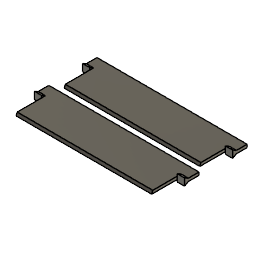
card-shuffler (Autodesk Fusion 360 archive; units mm, degrees)
design "card-shuffler-gates"
part number: 2026-07-29-22-33-21-616
part number: 2026-07-29-22-39-06-031
Autodesk Fusion 360 part; units mm, degrees
note: some values were not read from the file. Set by a fixed rule: which face or edge a step refers to.
(part 1 of 12)
sketch "Sketch1" plane through (0, 0, 0) normal (0, 0, 1) x (1, 0, 0)
  line L0 (0, 0) -> (93, 0)
  line L1 (93, 0) -> (93, -17.5)
  line L2 (93, -17.5) -> (0, -17.5)
  line L3 (0, -17.5) -> (0, 0)
  line L4 (93, 0) -> (98, 0)
  line L5 (93, -5) -> (93, 0)
  line L6 (0, 0) -> (-5, 0)
  line L7 (0, -15.5) -> (0, 0)
  line L8 (-5, 0) -> (98, 0)
  line L9 (98, 0) -> (98, 10)
  line L10 (98, 10) -> (-5, 10)
  line L11 (-5, 10) -> (-5, 0)
  line L12 (0, -15.5) -> (93, -15.5)
  line L13 (93, -15.5) -> (93, 10)
  line L14 (93, 10) -> (0, 10)
  line L15 (0, 10) -> (0, -15.5)
  dimension "d1" = 93
  dimension "d17" = 10
  dimension "d22" = 15.5
  dimension "d23" = 2
  constraint horizontal L0
  constraint vertical L1
  constraint horizontal L2
  constraint vertical L3
  constraint coincident L0.start L3.end
  constraint horizontal L4
  constraint vertical L5
  constraint horizontal L6
  constraint vertical L7
  constraint horizontal L8
  constraint vertical L9
  constraint horizontal L10
  constraint vertical L11
  constraint horizontal L12
  constraint vertical L13
  constraint horizontal L14
  constraint vertical L15
  constraint coincident L10 L13.end
  measures "d1" distance of L0.start L0.end
  measures "d17" distance of L6.end L10.end
  measures "d22" distance of L8 L12
  measures "d23" distance of L2 L12
extrude "Extrude1" add sketch "Sketch1" along normal blind 2 contours L6 L8 L10 L11 L15 | L4 L8 L9 L10 L13 makes body 1 at (-1.6667, 3.3333, 0) makes body 2 at (96.3333, 3.3333, 0)
extrude "Extrude3" add sketch "Sketch1" along normal blind 2 contours L0 L8 L10 L13 L14 L15 | L0 L1 L3 L5 L7 L8 L12 L13 L15 | L1 L2 L3 L12 bodies 1 2
sketch "Sketch3" plane through (0, 0, 0) normal (1, 0, 0) x (0, -1, 0)
  line L0 (-9, -5) -> (5, -5)
  line L1 (5, -5) -> (5, -2)
  line L2 (-9, -2) -> (16.216, -2) construction
  line L3 (5, -5) -> (10.1764, -5) construction
  line L4 (-9, -2) -> (-9, -5)
  line L5 (5, -2) -> (-9, -2)
  line L6 (0, 0) -> (17.5, 0)
  line L7 (17.5, 0) -> (17.5, -2)
  line L8 (17.5, -2) -> (0, -2)
  line L9 (17.5, 0) -> (16.7721, -2)
  line L10 (17.5, 0) -> (9.1284, 0) construction
  line L11 (0, -2) -> (0, 0)
  dimension "d16" = 110
  constraint horizontal L2
  constraint coincident L2.start L4.start
  constraint horizontal L3
  constraint coincident L0.end L1.start
  constraint horizontal L10
  constraint coincident L6.end L7.start
  constraint coincident L2 L9.end
  measures "d16" angle of L9 L10
extrude "Extrude2" cut sketch "Sketch3" along normal blind 95 contours L7 L8 L9 bodies 1
sketch "Sketch4" plane through (-5, 0, 0) normal (-1, 0, 0) x (0, -1, 0)
  line L0 (-10, 0) -> (0, 0)
  line L1 (0, 0) -> (0, 2)
  line L2 (0, 2) -> (-10, 2)
  line L3 (-10, 2) -> (-10, 0)
  line L4 (0, -1.5) -> (0, 3.5)
  line L5 (0, 3.5) -> (-4.3301, 1)
  line L6 (-4.3301, 1) -> (0, -1.5)
  point P0 (-1.4434, 1)
sketch "Sketch5" plane through (98, 0, 0) normal (1, 0, 0) x (0, 1, 0)
  line L0 (0, 0) -> (10, 0)
  line L1 (10, 0) -> (10, 2)
  line L2 (10, 2) -> (0, 2)
  line L3 (0, 2) -> (0, 0)
  line L4 (0, -1.5) -> (4.3301, 1)
  line L5 (4.3301, 1) -> (0, 3.5)
  line L6 (0, 3.5) -> (0, -1.5)
  point P0 (1.4434, 1)
extrude "Extrude4" add sketch "Sketch5" against normal blind 5 contours L0 L4 L6 | L2 L5 L6 bodies 1
extrude "Extrude5" add sketch "Sketch4" against normal blind 5 contours L0 L4 L6 | L2 L4 L5 bodies 1
copy_body "Body->Comp1" bodies 1 removing the originals makes body 3 in component "Component"
component "Component" placed x (1, 0, 0) y (0, 1, 0) z (0, 0, 1) at (0, 0, 0)
component "Component" placed x (1, 0, 0) y (0, 1, 0) z (0, 0, 1) at (0, 33, 0)
equation "d16 = 90 deg + 20 deg"

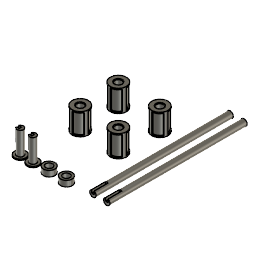
design "card-shuffler-wheels-and-shaft"
part number: 2026-07-30-19-48-15-416
part number: 2026-07-31-16-18-04-707
part number: 2026-07-31-16-25-10-615
part number: 2026-07-31-16-25-10-619
part number: 2026-08-15-23-04-46-105
part number: 2026-08-15-23-04-46-110
part number: 2026-08-17-15-33-29-178
Autodesk Fusion 360 part; units mm, degrees
sketch "Sketch4" plane through (0, 0, 0) normal (0, 0, 1) x (1, 0, 0)
  circle A0 centre (0, 0) radius 6
  circle A1 centre (0, 0) radius 7
  circle A2 centre (35, 0) radius 2.8
  circle A3 centre (0, 0) radius 7.5
  circle A4 centre (35, 0) radius 2.9
  line L0 (0, 0) -> (7, 0)
  line L1 (0, 0) -> (2.8348, 6.4003)
  line L2 (0, 0) -> (-7, 0) construction
  line L3 (0, 0) -> (-6.4003, 2.8348)
  line L4 (0, 0) -> (0, 7)
  line L5 (0, 0) -> (-2.8348, -6.4003)
  line L6 (0, 0) -> (-7, 0)
  line L7 (0, 0) -> (6.4003, -2.8348)
  line L8 (0, 0) -> (0, -7)
  circle A5 centre (0, -45) radius 5
  circle A6 centre (0, -45) radius 2.925
  circle A7 centre (-40, -45) radius 5
  line L9 (38, 1) -> (32, 1)
  line L10 (32, 1) -> (32, -1)
  line L11 (32, -1) -> (38, -1)
  line L12 (38, -1) -> (38, 1)
  line L13 (38, 1) -> (32, -1) construction
  line L14 (32, 1) -> (38, -1) construction
  line L15 (31.9, -1.1) -> (38.1, -1.1)
  line L16 (38.1, -1.1) -> (38.1, 1.1)
  line L17 (38.1, 1.1) -> (31.9, 1.1)
  line L18 (31.9, 1.1) -> (31.9, -1.1)
  line L19 (35, 1.1) -> (35, -1.1)
  line L20 (35.1, 1.1) -> (35.1, -1.1)
  point P0 (35, 0)
  dimension "d20" = 12
  dimension "d33" = 5.6
  dimension "d36" = 1
  dimension "d37" = 15
  dimension "d42" = 5.8
  dimension "d44" = 113.889
  dimension "d46" = 360
  dimension "d49" = 5.85
  dimension "d52" = 10
  dimension "d58" = 6
  dimension "d59" = 2
  dimension "d62" = 0.1
  constraint coincident A0.centre A1.centre
  constraint concentric A2 A4
  constraint coincident A1 L0.end
  constraint horizontal L0
  constraint horizontal L2
  constraint coincident A1 L1.end
  constraint concentric A5 A6
  constraint horizontal L9
  constraint perpendicular L9 L10
  constraint parallel L9 L11
  constraint parallel L10 L12
  constraint coincident L13 P0
  constraint coincident L14 P0
  constraint coincident P0 A2.centre
  constraint midpoint L17 L19.start
  constraint midpoint L15 L19.end
  constraint coincident L17 L20.start
  constraint coincident L15 L20.end
  constraint perpendicular L15 L20
  measures "d20" diameter of A0
  measures "d33" diameter of A2
  measures "d36" distance of A0 A1
  measures "d37" diameter of A3
  measures "d42" diameter of A4
  measures "d44" angle of L1 L2
  measures "d49" diameter of A6
  measures "d52" diameter of A7
  measures "d58" distance of L10.end L11.end
  measures "d59" distance of L9.end L10.end
extrude "Extrude3" add sketch "Sketch4" along normal blind 19 contours A0 L0 L1 | A0 L0 L7 | A0 L1 L4 | A0 L7 L8 | A0 L3 L6 | A0 L3 L4 | A0 L5 L8 | A0 L5 L6 makes body 1
sketch "Sketch5" plane through (0, 0, 19) normal (0, 0, 1) x (-1, 0, 0)
  circle A0 centre (0, 0) radius 6
  circle A1 centre (0, 0) radius 7
  circle A2 centre (0, 0) radius 2.925
  dimension "d24" = 14
  dimension "d29" = 5.85
  constraint coincident A0.centre A1.centre
  measures "d24" diameter of A1
  measures "d29" diameter of A2
extrude "Extrude5" add sketch "Sketch5" against normal blind 1 contours A1 bodies 1
extrude "Extrude4" add sketch "Sketch4" along normal blind 1 contours A0 A1 L0 L7 | A0 A1 L0 L1 | A0 A1 L1 L4 | A0 A1 L7 L8 | A0 A1 L3 L4 | A0 A1 L5 L8 | A0 A1 L3 L6 | A0 A1 L5 L6 bodies 1
extrude "Extrude6" cut sketch "Sketch5" against normal blind 19 contours A2 bodies 1
chamfer "Chamfer1" distance 0.5 angle 45 2 edges at (2.7271, 1.0577, 0) (2.7271, -1.0577, 19) on bodies 1
extrude "Extrude9" add sketch "Sketch4" along normal blind 19 contours A0 A1 L0 L7 | A0 A1 L1 L4 | A0 A1 L5 L8 | A0 A1 L3 L6 bodies 1
copy_body "Body->Comp2" bodies 1 removing the originals makes body 2 in component "Component"
extrude "Extrude7" add sketch "Sketch4" along normal blind 119 separate body contours A2 L9 L11 L20 | A2 L9 L17 L20 | A2 L11 L15 L20 | A2 L17 | L9 L11 L19 L20 | L9 L17 L19 L20 | A2 L15 | L11 L15 L19 L20 | A2 L9 L17 L19 | A2 L9 L11 L19 | A2 L11 L15 L19 makes body 3
extrude "Extrude13" cut sketch "Sketch4" along normal blind 12 contours L9 L11 L19 L20 | L9 L17 L19 L20 | L11 L15 L19 L20 | A2 L9 L17 L19 | A2 L9 L11 L19 | A2 L11 L15 L19 bodies 3
copy_body "CopyPasteBodies1" bodies 3 makes body 4
move_body "Move1" bodies 4 to x (1, 0, 0) y (0, 1, 0) z (0, 0, 1) at (-12, 0, 0)
copy_body "Body->Comp3" bodies 3 removing the originals makes body 5 in component "Component'"
copy_body "Body->Comp4" bodies 4 removing the originals makes body 6 in component "Component''"
move_body "Move1'" bodies 6 to x (1, 0, 0) y (0, 0, -1) z (0, 1, 0) at (0, -45, 3) in component "Component''"
move_body "Move1''" bodies 5 to x (1, 0, 0) y (0, 0, -1) z (0, 1, 0) at (0, -45, 3) in component "Component'"
extrude "Extrude10" add sketch "Sketch4" along normal blind 5 separate body contours A5 makes body 7
copy_body "CopyPasteBodies3" bodies 7 makes body 8
move_body "Move4" bodies 8 to x (1, 0, 0) y (0, 1, 0) z (0, 0, 1) at (-15, 0, 0)
copy_body "Body->Comp7" bodies 8 removing the originals makes body 9 in component "Component'''"
copy_body "Body->Comp8" bodies 7 removing the originals makes body 10 in component "Component''''"
extrude "Extrude11" add sketch "Sketch4" along normal blind 1 separate body contours A7 makes body 11
sketch "Sketch6" plane through (0, 0, 1) normal (0, 0, 1) x (-1, 0, 0)
  circle A0 centre (40, 45) radius 5
  circle A1 centre (40, 45) radius 2.8
  line L0 (37, 44) -> (43, 44)
  line L1 (43, 44) -> (43, 46)
  line L2 (43, 46) -> (37, 46)
  line L3 (37, 46) -> (37, 44)
  line L4 (37, 44) -> (43, 46) construction
  line L5 (43, 44) -> (37, 46) construction
  line L6 (40, 44) -> (40, 46)
  line L7 (39.9, 44) -> (39.9, 46)
  point P0 (40, 45)
  dimension "d55" = 5.6
  constraint concentric A0 A1
  constraint horizontal L0
  constraint perpendicular L0 L1
  constraint parallel L0 L2
  constraint parallel L1 L3
  constraint coincident L4 P0
  constraint coincident L5 P0
  constraint coincident P0 A0.centre
  constraint midpoint L0 L6.start
  constraint midpoint L2 L6.end
  constraint coincident L0 L7.start
  constraint coincident L2 L7.end
  constraint perpendicular L2 L7
  measures "d55" diameter of A1
extrude "Extrude12" add sketch "Sketch6" along normal blind 20 contours A1 L2 | A1 L0 | A1 L0 L2 L7 bodies 11
extrude "Extrude14" add sketch "Sketch6" along normal blind 8 contours A1 L0 L2 L6 bodies 11
copy_body "Body->Comp9" bodies 11 removing the originals makes body 12 in component "Component'''''"
component "Component" placed x (1, 0, 0) y (0, 1, 0) z (0, 0, 1) at (0, 0, 0)
component "Component" placed x (1, 0, 0) y (0, 1, 0) z (0, 0, 1) at (-33, 0, 0)
component "Component" placed x (1, 0, 0) y (0, 1, 0) z (0, 0, 1) at (-34, 34, 0)
component "Component" placed x (1, 0, 0) y (0, 1, 0) z (0, 0, 1) at (2, 34, 0)
component "Component'" placed x (0, 0, -1) y (0, 1, 0) z (1, 0, 0) at (31.9518, 0, 37.9518)
component "Component''" placed x (0, 0, -1) y (0, 1, 0) z (1, 0, 0) at (19.9518, 0, 25.9518)
component "Component'''" placed x (1, 0, 0) y (0, 1, 0) z (0, 0, 1) at (0, 0, 0)
component "Component''''" placed x (1, 0, 0) y (0, 1, 0) z (0, 0, 1) at (0, 0, 0)
component "Component'''''" placed x (1, 0, 0) y (0, 1, 0) z (0, 0, 1) at (0, 0, 0)
component "Component'''''" placed x (1, 0, 0) y (0, 1, 0) z (0, 0, 1) at (11, 0, 0)
equation "d34 = 93 mm + 20 mm + 6 mm"
equation "d44 = 180 deg - 66.11051484 deg"

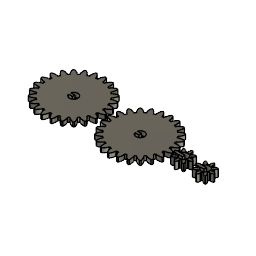
design "card-shuffler-middle-gears"
part number: 2026-08-17-02-18-25-515
part number: 2026-08-18-19-56-53-081
part number: 2026-08-18-20-31-36-499
Autodesk Fusion 360 part; units mm, degrees
sketch "Sketch1" plane through (0, 0, 0) normal (0, 0, 1) x (1, 0, 0) in component "Component"
  spline S0 degree 5 poles (4.4841, -1.024) (4.4842, -1.0241) (4.4844, -1.0241) (4.4848, -1.0242) (4.4853, -1.0243) (4.486, -1.0244) (4.4869, -1.0246) (4.4879, -1.0248) (4.489, -1.025) (4.4903, -1.0252) (4.4916, -1.0254) (4.4931, -1.0257) (4.4947, -1.0259) (4.4963, -1.0262) (4.4981, -1.0264) (4.5, -1.0267) (4.502, -1.027) (4.5042, -1.0272) (4.5064, -1.0275) (4.5087, -1.0278) (4.5111, -1.0281) (4.5136, -1.0284) (4.5162, -1.0287) (4.5189, -1.0289) (4.5218, -1.0292) (4.5247, -1.0295) (4.5277, -1.0297) (4.5308, -1.03) (4.534, -1.0302) (4.5372, -1.0305) (4.5406, -1.0307) (4.5441, -1.0309) (4.5476, -1.0311) (4.5513, -1.0313) (4.555, -1.0315) (4.5588, -1.0317) (4.5627, -1.0319) (4.5667, -1.032) (4.5708, -1.0321) (4.575, -1.0322) (4.5792, -1.0323) (4.5835, -1.0324) (4.5879, -1.0325) (4.5924, -1.0325) (4.597, -1.0325) (4.6016, -1.0325) (4.6064, -1.0325) (4.6111, -1.0324) (4.616, -1.0324) (4.621, -1.0323) (4.626, -1.0322) (4.6311, -1.032) (4.6363, -1.0319) (4.6415, -1.0317) (4.6468, -1.0315) (4.6522, -1.0312) (4.6577, -1.031) (4.6632, -1.0307) (4.6688, -1.0303) (4.6745, -1.03) (4.6802, -1.0296) (4.686, -1.0292) (4.6919, -1.0288) (4.6978, -1.0283) (4.7038, -1.0278) (4.7099, -1.0272) (4.716, -1.0267) (4.7222, -1.0261) (4.7285, -1.0255) (4.7348, -1.0248) (4.7412, -1.0241) (4.7476, -1.0234) (4.7541, -1.0226) (4.7607, -1.0218) (4.7673, -1.021) (4.774, -1.0201) (4.7807, -1.0192) (4.7875, -1.0182) (4.7944, -1.0173) (4.8013, -1.0162) (4.8083, -1.0152) (4.8153, -1.0141) (4.8224, -1.013) (4.8295, -1.0118) (4.8367, -1.0106) (4.8439, -1.0093) (4.8512, -1.0081) (4.8585, -1.0067) (4.8659, -1.0054) (4.8734, -1.004) (4.8809, -1.0025) (4.8884, -1.001) (4.896, -0.9995) (4.9037, -0.9979) (4.9114, -0.9963) (4.9191, -0.9947) (4.9269, -0.993) (4.9347, -0.9912) (4.9426, -0.9894) (4.9505, -0.9876) (4.9585, -0.9858) (4.9665, -0.9838) (4.9746, -0.9819) (4.9827, -0.9799) (4.9908, -0.9778) (4.999, -0.9757) (5.0073, -0.9736) (5.0155, -0.9714) (5.0239, -0.9692) (5.0322, -0.9669) (5.0406, -0.9646) (5.0491, -0.9623) (5.0576, -0.9599) (5.0661, -0.9574) (5.0746, -0.9549) (5.0832, -0.9524) (5.0919, -0.9498) (5.1005, -0.9471) (5.1092, -0.9444) (5.118, -0.9417) (5.1268, -0.9389) (5.1356, -0.9361) (5.1444, -0.9332) (5.1533, -0.9303) (5.1623, -0.9273) (5.1712, -0.9243) (5.1802, -0.9212) (5.1892, -0.9181) (5.1983, -0.9149) (5.2074, -0.9117) (5.2165, -0.9084) (5.2256, -0.9051) (5.2348, -0.9017) (5.244, -0.8983) (5.2533, -0.8948) (5.2626, -0.8913) (5.2719, -0.8877) (5.2812, -0.8841) (5.2905, -0.8804) (5.2999, -0.8767) (5.3094, -0.8729) (5.3188, -0.8691) (5.3283, -0.8652) (5.3378, -0.8613) (5.3473, -0.8573) (5.3568, -0.8533) (5.3664, -0.8492) (5.376, -0.8451) (5.3856, -0.8409) (5.3953, -0.8367) (5.4049, -0.8324) (5.4146, -0.8281) (5.4244, -0.8237) (5.4341, -0.8192) (5.4439, -0.8147) (5.4537, -0.8102) (5.4635, -0.8056) (5.4733, -0.8009) (5.4831, -0.7962) (5.493, -0.7915) (5.5029, -0.7867) (5.5128, -0.7818) (5.5227, -0.7769) (5.5327, -0.7719) (5.5426, -0.7669) (5.5526, -0.7618) (5.5626, -0.7567) (5.5726, -0.7515) (5.5827, -0.7463) (5.5927, -0.741) (5.6028, -0.7356) (5.6129, -0.7302) (5.623, -0.7248) (5.6331, -0.7193) (5.6432, -0.7137) (5.6534, -0.7081) (5.6636, -0.7024) (5.6737, -0.6967) (5.6839, -0.6909) (5.6941, -0.6851) (5.7043, -0.6792) (5.7146, -0.6733) (5.7248, -0.6673) (5.7351, -0.6613) (5.7453, -0.6552) (5.7556, -0.649) (5.7659, -0.6428) (5.7762, -0.6365) (5.7865, -0.6302) (5.7968, -0.6239) (5.8071, -0.6174) (5.8175, -0.611) (5.8278, -0.6044) (5.8382, -0.5978) (5.8485, -0.5912) (5.8589, -0.5845) (5.8693, -0.5777) (5.8797, -0.5709) (5.8901, -0.5641) (5.9005, -0.5572) (5.9109, -0.5502) (5.9213, -0.5432) (5.9317, -0.5361) (5.9421, -0.529) (5.9525, -0.5218) (5.963, -0.5145) (5.9734, -0.5072) (5.9839, -0.4999) (5.9943, -0.4925) (6.0048, -0.485) (6.0152, -0.4775) (6.0257, -0.4699) (6.0361, -0.4623) (6.0466, -0.4546) (6.057, -0.4469) (6.0675, -0.4391) (6.078, -0.4313) (6.0884, -0.4234) (6.0989, -0.4154) (6.1094, -0.4074) (6.1199, -0.3993) (6.1303, -0.3912) (6.1408, -0.383) (6.1513, -0.3748) (6.1617, -0.3665) (6.1722, -0.3582) (6.1827, -0.3498) (6.1931, -0.3414) (6.2036, -0.3329) (6.2141, -0.3243) (6.2245, -0.3157) (6.235, -0.3071) (6.2454, -0.2983) (6.2559, -0.2896) (6.2663, -0.2807) (6.2768, -0.2719) (6.2872, -0.2629) (6.2976, -0.2539) (6.3081, -0.2449) (6.3185, -0.2358) (6.3289, -0.2267) (6.3372, -0.2193) (6.3435, -0.2137) (6.3476, -0.21) (6.3497, -0.2082) knots 0 0 0 0 0 0 0.00416667 0.00833333 0.0125 0.01666667 0.02083333 0.025 0.02916667 0.03333333 0.0375 0.04166667 0.04583333 0.05 0.05416667 0.05833333 0.0625 0.06666667 0.07083333 0.075 0.07916667 0.08333333 0.0875 0.09166667 0.09583333 0.1 0.10416667 0.10833333 0.1125 0.11666667 0.12083333 0.125 0.12916667 0.13333333 0.1375 0.14166667 0.14583333 0.15 0.15416667 0.15833333 0.1625 0.16666667 0.17083333 0.175 0.17916667 0.18333333 0.1875 0.19166667 0.19583333 0.2 0.20416667 0.20833333 0.2125 0.21666667 0.22083333 0.225 0.22916667 0.23333333 0.2375 0.24166667 0.24583333 0.25 0.25416667 0.25833333 0.2625 0.26666667 0.27083333 0.275 0.27916667 0.28333333 0.2875 0.29166667 0.29583333 0.3 0.30416667 0.30833333 0.3125 0.31666667 0.32083333 0.325 0.32916667 0.33333333 0.3375 0.34166667 0.34583333 0.35 0.35416667 0.35833333 0.3625 0.36666667 0.37083333 0.375 0.37916667 0.38333333 0.3875 0.39166667 0.39583333 0.4 0.40416667 0.40833333 0.4125 0.41666667 0.42083333 0.425 0.42916667 0.43333333 0.4375 0.44166667 0.44583333 0.45 0.45416667 0.45833333 0.4625 0.46666667 0.47083333 0.475 0.47916667 0.48333333 0.4875 0.49166667 0.49583333 0.5 0.50416667 0.50833333 0.5125 0.51666667 0.52083333 0.525 0.52916667 0.53333333 0.5375 0.54166667 0.54583333 0.55 0.55416667 0.55833333 0.5625 0.56666667 0.57083333 0.575 0.57916667 0.58333333 0.5875 0.59166667 0.59583333 0.6 0.60416667 0.60833333 0.6125 0.61666667 0.62083333 0.625 0.62916667 0.63333333 0.6375 0.64166667 0.64583333 0.65 0.65416667 0.65833333 0.6625 0.66666667 0.67083333 0.675 0.67916667 0.68333333 0.6875 0.69166667 0.69583333 0.7 0.70416667 0.70833333 0.7125 0.71666667 0.72083333 0.725 0.72916667 0.73333333 0.7375 0.74166667 0.74583333 0.75 0.75416667 0.75833333 0.7625 0.76666667 0.77083333 0.775 0.77916667 0.78333333 0.7875 0.79166667 0.79583333 0.8 0.80416667 0.80833333 0.8125 0.81666667 0.82083333 0.825 0.82916667 0.83333333 0.8375 0.84166667 0.84583333 0.85 0.85416667 0.85833333 0.8625 0.86666667 0.87083333 0.875 0.87916667 0.88333333 0.8875 0.89166667 0.89583333 0.9 0.90416667 0.90833333 0.9125 0.91666667 0.92083333 0.925 0.92916667 0.93333333 0.9375 0.94166667 0.94583333 0.95 0.95416667 0.95833333 0.9625 0.96666667 0.97083333 0.975 0.97916667 0.98333333 0.9875 0.99166667 0.99583333 1 1 1 1 1 1
  spline S1 degree 5 poles (4.4841, 1.024) (4.4842, 1.0241) (4.4844, 1.0241) (4.4848, 1.0242) (4.4853, 1.0243) (4.486, 1.0244) (4.4869, 1.0246) (4.4879, 1.0248) (4.489, 1.025) (4.4903, 1.0252) (4.4916, 1.0254) (4.4931, 1.0257) (4.4947, 1.0259) (4.4963, 1.0262) (4.4981, 1.0264) (4.5, 1.0267) (4.502, 1.027) (4.5042, 1.0272) (4.5064, 1.0275) (4.5087, 1.0278) (4.5111, 1.0281) (4.5136, 1.0284) (4.5162, 1.0287) (4.5189, 1.0289) (4.5218, 1.0292) (4.5247, 1.0295) (4.5277, 1.0297) (4.5308, 1.03) (4.534, 1.0302) (4.5372, 1.0305) (4.5406, 1.0307) (4.5441, 1.0309) (4.5476, 1.0311) (4.5513, 1.0313) (4.555, 1.0315) (4.5588, 1.0317) (4.5627, 1.0319) (4.5667, 1.032) (4.5708, 1.0321) (4.575, 1.0322) (4.5792, 1.0323) (4.5835, 1.0324) (4.5879, 1.0325) (4.5924, 1.0325) (4.597, 1.0325) (4.6016, 1.0325) (4.6064, 1.0325) (4.6111, 1.0324) (4.616, 1.0324) (4.621, 1.0323) (4.626, 1.0322) (4.6311, 1.032) (4.6363, 1.0319) (4.6415, 1.0317) (4.6468, 1.0315) (4.6522, 1.0312) (4.6577, 1.031) (4.6632, 1.0307) (4.6688, 1.0303) (4.6745, 1.03) (4.6802, 1.0296) (4.686, 1.0292) (4.6919, 1.0288) (4.6978, 1.0283) (4.7038, 1.0278) (4.7099, 1.0272) (4.716, 1.0267) (4.7222, 1.0261) (4.7285, 1.0255) (4.7348, 1.0248) (4.7412, 1.0241) (4.7476, 1.0234) (4.7541, 1.0226) (4.7607, 1.0218) (4.7673, 1.021) (4.774, 1.0201) (4.7807, 1.0192) (4.7875, 1.0182) (4.7944, 1.0173) (4.8013, 1.0162) (4.8083, 1.0152) (4.8153, 1.0141) (4.8224, 1.013) (4.8295, 1.0118) (4.8367, 1.0106) (4.8439, 1.0093) (4.8512, 1.0081) (4.8585, 1.0067) (4.8659, 1.0054) (4.8734, 1.004) (4.8809, 1.0025) (4.8884, 1.001) (4.896, 0.9995) (4.9037, 0.9979) (4.9114, 0.9963) (4.9191, 0.9947) (4.9269, 0.993) (4.9347, 0.9912) (4.9426, 0.9894) (4.9505, 0.9876) (4.9585, 0.9858) (4.9665, 0.9838) (4.9746, 0.9819) (4.9827, 0.9799) (4.9908, 0.9778) (4.999, 0.9757) (5.0073, 0.9736) (5.0155, 0.9714) (5.0239, 0.9692) (5.0322, 0.9669) (5.0406, 0.9646) (5.0491, 0.9623) (5.0576, 0.9599) (5.0661, 0.9574) (5.0746, 0.9549) (5.0832, 0.9524) (5.0919, 0.9498) (5.1005, 0.9471) (5.1092, 0.9444) (5.118, 0.9417) (5.1268, 0.9389) (5.1356, 0.9361) (5.1444, 0.9332) (5.1533, 0.9303) (5.1623, 0.9273) (5.1712, 0.9243) (5.1802, 0.9212) (5.1892, 0.9181) (5.1983, 0.9149) (5.2074, 0.9117) (5.2165, 0.9084) (5.2256, 0.9051) (5.2348, 0.9017) (5.244, 0.8983) (5.2533, 0.8948) (5.2626, 0.8913) (5.2719, 0.8877) (5.2812, 0.8841) (5.2905, 0.8804) (5.2999, 0.8767) (5.3094, 0.8729) (5.3188, 0.8691) (5.3283, 0.8652) (5.3378, 0.8613) (5.3473, 0.8573) (5.3568, 0.8533) (5.3664, 0.8492) (5.376, 0.8451) (5.3856, 0.8409) (5.3953, 0.8367) (5.4049, 0.8324) (5.4146, 0.8281) (5.4244, 0.8237) (5.4341, 0.8192) (5.4439, 0.8147) (5.4537, 0.8102) (5.4635, 0.8056) (5.4733, 0.8009) (5.4831, 0.7962) (5.493, 0.7915) (5.5029, 0.7867) (5.5128, 0.7818) (5.5227, 0.7769) (5.5327, 0.7719) (5.5426, 0.7669) (5.5526, 0.7618) (5.5626, 0.7567) (5.5726, 0.7515) (5.5827, 0.7463) (5.5927, 0.741) (5.6028, 0.7356) (5.6129, 0.7302) (5.623, 0.7248) (5.6331, 0.7193) (5.6432, 0.7137) (5.6534, 0.7081) (5.6636, 0.7024) (5.6737, 0.6967) (5.6839, 0.6909) (5.6941, 0.6851) (5.7043, 0.6792) (5.7146, 0.6733) (5.7248, 0.6673) (5.7351, 0.6613) (5.7453, 0.6552) (5.7556, 0.649) (5.7659, 0.6428) (5.7762, 0.6365) (5.7865, 0.6302) (5.7968, 0.6239) (5.8071, 0.6174) (5.8175, 0.611) (5.8278, 0.6044) (5.8382, 0.5978) (5.8485, 0.5912) (5.8589, 0.5845) (5.8693, 0.5777) (5.8797, 0.5709) (5.8901, 0.5641) (5.9005, 0.5572) (5.9109, 0.5502) (5.9213, 0.5432) (5.9317, 0.5361) (5.9421, 0.529) (5.9525, 0.5218) (5.963, 0.5145) (5.9734, 0.5072) (5.9839, 0.4999) (5.9943, 0.4925) (6.0048, 0.485) (6.0152, 0.4775) (6.0257, 0.4699) (6.0361, 0.4623) (6.0466, 0.4546) (6.057, 0.4469) (6.0675, 0.4391) (6.078, 0.4313) (6.0884, 0.4234) (6.0989, 0.4154) (6.1094, 0.4074) (6.1199, 0.3993) (6.1303, 0.3912) (6.1408, 0.383) (6.1513, 0.3748) (6.1617, 0.3665) (6.1722, 0.3582) (6.1827, 0.3498) (6.1931, 0.3414) (6.2036, 0.3329) (6.2141, 0.3243) (6.2245, 0.3157) (6.235, 0.3071) (6.2454, 0.2983) (6.2559, 0.2896) (6.2663, 0.2807) (6.2768, 0.2719) (6.2872, 0.2629) (6.2976, 0.2539) (6.3081, 0.2449) (6.3185, 0.2358) (6.3289, 0.2267) (6.3372, 0.2193) (6.3435, 0.2137) (6.3476, 0.21) (6.3497, 0.2082) knots 0 0 0 0 0 0 0.00416667 0.00833333 0.0125 0.01666667 0.02083333 0.025 0.02916667 0.03333333 0.0375 0.04166667 0.04583333 0.05 0.05416667 0.05833333 0.0625 0.06666667 0.07083333 0.075 0.07916667 0.08333333 0.0875 0.09166667 0.09583333 0.1 0.10416667 0.10833333 0.1125 0.11666667 0.12083333 0.125 0.12916667 0.13333333 0.1375 0.14166667 0.14583333 0.15 0.15416667 0.15833333 0.1625 0.16666667 0.17083333 0.175 0.17916667 0.18333333 0.1875 0.19166667 0.19583333 0.2 0.20416667 0.20833333 0.2125 0.21666667 0.22083333 0.225 0.22916667 0.23333333 0.2375 0.24166667 0.24583333 0.25 0.25416667 0.25833333 0.2625 0.26666667 0.27083333 0.275 0.27916667 0.28333333 0.2875 0.29166667 0.29583333 0.3 0.30416667 0.30833333 0.3125 0.31666667 0.32083333 0.325 0.32916667 0.33333333 0.3375 0.34166667 0.34583333 0.35 0.35416667 0.35833333 0.3625 0.36666667 0.37083333 0.375 0.37916667 0.38333333 0.3875 0.39166667 0.39583333 0.4 0.40416667 0.40833333 0.4125 0.41666667 0.42083333 0.425 0.42916667 0.43333333 0.4375 0.44166667 0.44583333 0.45 0.45416667 0.45833333 0.4625 0.46666667 0.47083333 0.475 0.47916667 0.48333333 0.4875 0.49166667 0.49583333 0.5 0.50416667 0.50833333 0.5125 0.51666667 0.52083333 0.525 0.52916667 0.53333333 0.5375 0.54166667 0.54583333 0.55 0.55416667 0.55833333 0.5625 0.56666667 0.57083333 0.575 0.57916667 0.58333333 0.5875 0.59166667 0.59583333 0.6 0.60416667 0.60833333 0.6125 0.61666667 0.62083333 0.625 0.62916667 0.63333333 0.6375 0.64166667 0.64583333 0.65 0.65416667 0.65833333 0.6625 0.66666667 0.67083333 0.675 0.67916667 0.68333333 0.6875 0.69166667 0.69583333 0.7 0.70416667 0.70833333 0.7125 0.71666667 0.72083333 0.725 0.72916667 0.73333333 0.7375 0.74166667 0.74583333 0.75 0.75416667 0.75833333 0.7625 0.76666667 0.77083333 0.775 0.77916667 0.78333333 0.7875 0.79166667 0.79583333 0.8 0.80416667 0.80833333 0.8125 0.81666667 0.82083333 0.825 0.82916667 0.83333333 0.8375 0.84166667 0.84583333 0.85 0.85416667 0.85833333 0.8625 0.86666667 0.87083333 0.875 0.87916667 0.88333333 0.8875 0.89166667 0.89583333 0.9 0.90416667 0.90833333 0.9125 0.91666667 0.92083333 0.925 0.92916667 0.93333333 0.9375 0.94166667 0.94583333 0.95 0.95416667 0.95833333 0.9625 0.96666667 0.97083333 0.975 0.97916667 0.98333333 0.9875 0.99166667 0.99583333 1 1 1 1 1 1
  spline S2 degree 5 poles (4.4833, -1.0239) (4.4833, -1.0239) (4.4834, -1.0239) (4.4835, -1.0239) (4.4836, -1.0239) (4.4838, -1.024) (4.4839, -1.024) (4.484, -1.024) (4.4841, -1.024) (4.4841, -1.024) knots 0 0 0 0 0 0 0.2 0.4 0.6 0.8 1 1 1 1 1 1
  spline S3 degree 5 poles (4.4833, 1.0239) (4.4833, 1.0239) (4.4834, 1.0239) (4.4835, 1.0239) (4.4836, 1.0239) (4.4838, 1.024) (4.4839, 1.024) (4.484, 1.024) (4.4841, 1.024) (4.4841, 1.024) knots 0 0 0 0 0 0 0.2 0.4 0.6 0.8 1 1 1 1 1 1
  line L0 (0, 0) -> (4.4833, -1.0239)
  line L1 (0, 0) -> (4.4833, 1.0239)
  arc A0 (6.3497, -0.2082) -> (6.3497, 0.2082) centre (0, 0) ccw
  point P0 (4.4867, -1.0245)
  point P1 (4.491, -1.0253)
  point P2 (4.497, -1.0263)
  point P3 (4.5047, -1.0273)
  point P4 (4.5143, -1.0284)
  point P5 (4.5255, -1.0295)
  point P6 (4.5385, -1.0306)
  point P7 (4.5533, -1.0314)
  point P8 (4.5698, -1.0321)
  point P9 (4.5881, -1.0325)
  point P10 (4.6081, -1.0325)
  point P11 (4.6298, -1.0321)
  point P12 (4.6533, -1.0312)
  point P13 (4.6785, -1.0297)
  point P14 (4.7054, -1.0276)
  point P15 (4.734, -1.0249)
  point P16 (4.7642, -1.0213)
  point P17 (4.7961, -1.017)
  point P18 (4.8296, -1.0118)
  point P19 (4.8648, -1.0056)
  point P20 (4.9015, -0.9984)
  point P21 (4.9398, -0.9901)
  point P22 (4.9795, -0.9807)
  point P23 (5.0208, -0.97)
  point P24 (5.0636, -0.9581)
  point P25 (5.1078, -0.9449)
  point P26 (5.1533, -0.9303)
  point P27 (5.2002, -0.9142)
  point P28 (5.2485, -0.8966)
  point P29 (5.298, -0.8775)
  point P30 (5.3487, -0.8567)
  point P31 (5.4006, -0.8343)
  point P32 (5.4537, -0.8102)
  point P33 (5.5078, -0.7842)
  point P34 (5.563, -0.7565)
  point P35 (5.6192, -0.7268)
  point P36 (5.6763, -0.6953)
  point P37 (5.7343, -0.6617)
  point P38 (5.7931, -0.6261)
  point P39 (5.8527, -0.5885)
  point P40 (5.913, -0.5488)
  point P41 (5.9739, -0.5069)
  point P42 (6.0355, -0.4628)
  point P43 (6.0975, -0.4165)
  point P44 (6.16, -0.3679)
  point P45 (6.223, -0.317)
  point P46 (6.2862, -0.2638)
  point P47 (4.4867, 1.0245)
  point P48 (4.491, 1.0253)
  point P49 (4.497, 1.0263)
  point P50 (4.5047, 1.0273)
  point P51 (4.5143, 1.0284)
  point P52 (4.5255, 1.0295)
  point P53 (4.5385, 1.0306)
  point P54 (4.5533, 1.0314)
  point P55 (4.5698, 1.0321)
  point P56 (4.5881, 1.0325)
  point P57 (4.6081, 1.0325)
  point P58 (4.6298, 1.0321)
  point P59 (4.6533, 1.0312)
  point P60 (4.6785, 1.0297)
  point P61 (4.7054, 1.0276)
  point P62 (4.734, 1.0249)
  point P63 (4.7642, 1.0213)
  point P64 (4.7961, 1.017)
  point P65 (4.8296, 1.0118)
  point P66 (4.8648, 1.0056)
  point P67 (4.9015, 0.9984)
  point P68 (4.9398, 0.9901)
  point P69 (4.9795, 0.9807)
  point P70 (5.0208, 0.97)
  point P71 (5.0636, 0.9581)
  point P72 (5.1078, 0.9449)
  point P73 (5.1533, 0.9303)
  point P74 (5.2002, 0.9142)
  point P75 (5.2485, 0.8966)
  point P76 (5.298, 0.8775)
  point P77 (5.3487, 0.8567)
  point P78 (5.4006, 0.8343)
  point P79 (5.4537, 0.8102)
  point P80 (5.5078, 0.7842)
  point P81 (5.563, 0.7565)
  point P82 (5.6192, 0.7268)
  point P83 (5.6763, 0.6953)
  point P84 (5.7343, 0.6617)
  point P85 (5.7931, 0.6261)
  point P86 (5.8527, 0.5885)
  point P87 (5.913, 0.5488)
  point P88 (5.9739, 0.5069)
  point P89 (6.0355, 0.4628)
  point P90 (6.0975, 0.4165)
  point P91 (6.16, 0.3679)
  point P92 (6.223, 0.317)
  point P93 (6.2862, 0.2638)
sketch "Sketch2" plane through (0, 0, 0) normal (0, 0, 1) x (1, 0, 0) in component "Component"
  circle A0 centre (0, 0) radius 3.6813
extrude "Extrude1" add sketch "Sketch2" along normal blind 5 makes body 1 in component "Component"
extrude "Extrude2" add sketch "Sketch1" along normal blind 5 separate body makes body 2 in component "Component"
pattern_circular "C-Pattern1" count 8 over 360 about axis through (0, 0, 1.75) along (0, 0, 1) of "Extrude2" makes body 3 at (1.2983, 0.8155, 1.6667) makes body 4 at (0.3413, 1.4947, 1.6667) makes body 5 at (-0.8155, 1.2983, 1.6667) makes body 6 at (-1.4947, 0.3413, 1.6667) makes body 7 at (-1.2983, -0.8155, 1.6667) makes body 8 at (-0.3413, -1.4947, 1.6667) makes body 9 at (0.8155, -1.2983, 1.6667) in component "Component"
sketch "Sketch3" plane through (0, 0, 0) normal (0, 0, 1) x (1, 0, 0) in component "Component"
  line L0 (0, 0) -> (51.0366, 0) construction
  line L1 (51.0366, 0) -> (51.0366, 3) construction
  line L2 (51.0366, 3) -> (0, 3) construction
  line L3 (0, 3) -> (0, 0) construction
  constraint perpendicular L0 L1
  constraint parallel L0 L2
  constraint parallel L1 L3
combine "Combine1" operation add target body 1 tool bodies 2 3 4 5 6 7 8 9 in component "Component"
sketch "Sketch1 (2)" plane through (0, 0, 0) normal (0, 0, 1) x (1, 0, 0) in component "Component'"
  spline S0 degree 5 poles (18.5341, -1.774) (18.5343, -1.774) (18.5348, -1.7741) (18.5356, -1.7741) (18.5368, -1.7742) (18.5386, -1.7743) (18.5407, -1.7745) (18.5432, -1.7746) (18.5459, -1.7748) (18.5489, -1.775) (18.5521, -1.7751) (18.5556, -1.7753) (18.5594, -1.7755) (18.5634, -1.7756) (18.5676, -1.7758) (18.5721, -1.7759) (18.5768, -1.776) (18.5818, -1.7762) (18.587, -1.7763) (18.5924, -1.7764) (18.598, -1.7764) (18.6038, -1.7765) (18.6098, -1.7765) (18.616, -1.7766) (18.6224, -1.7765) (18.629, -1.7765) (18.6358, -1.7765) (18.6428, -1.7764) (18.65, -1.7763) (18.6574, -1.7761) (18.6649, -1.776) (18.6726, -1.7758) (18.6805, -1.7755) (18.6885, -1.7753) (18.6968, -1.775) (18.7051, -1.7747) (18.7137, -1.7743) (18.7224, -1.7739) (18.7313, -1.7735) (18.7403, -1.773) (18.7495, -1.7725) (18.7588, -1.7719) (18.7683, -1.7713) (18.7779, -1.7707) (18.7876, -1.77) (18.7975, -1.7693) (18.8076, -1.7686) (18.8178, -1.7678) (18.8281, -1.7669) (18.8386, -1.766) (18.8492, -1.7651) (18.8599, -1.7641) (18.8707, -1.7631) (18.8817, -1.762) (18.8928, -1.7609) (18.9041, -1.7598) (18.9154, -1.7586) (18.9269, -1.7573) (18.9385, -1.756) (18.9502, -1.7546) (18.9621, -1.7532) (18.974, -1.7518) (18.9861, -1.7503) (18.9983, -1.7487) (19.0106, -1.7471) (19.023, -1.7454) (19.0355, -1.7437) (19.0481, -1.742) (19.0609, -1.7401) (19.0737, -1.7383) (19.0867, -1.7363) (19.0997, -1.7344) (19.1129, -1.7323) (19.1261, -1.7302) (19.1395, -1.7281) (19.1529, -1.7259) (19.1665, -1.7237) (19.1801, -1.7213) (19.1939, -1.719) (19.2077, -1.7166) (19.2217, -1.7141) (19.2357, -1.7115) (19.2498, -1.7089) (19.2641, -1.7063) (19.2784, -1.7036) (19.2928, -1.7008) (19.3072, -1.698) (19.3218, -1.6951) (19.3365, -1.6921) (19.3512, -1.6891) (19.3661, -1.6861) (19.381, -1.683) (19.396, -1.6798) (19.4111, -1.6765) (19.4262, -1.6732) (19.4415, -1.6699) (19.4568, -1.6664) (19.4722, -1.663) (19.4877, -1.6594) (19.5033, -1.6558) (19.5189, -1.6521) (19.5346, -1.6484) (19.5504, -1.6446) (19.5663, -1.6407) (19.5822, -1.6368) (19.5982, -1.6328) (19.6143, -1.6288) (19.6305, -1.6247) (19.6467, -1.6205) (19.663, -1.6163) (19.6794, -1.612) (19.6958, -1.6076) (19.7123, -1.6032) (19.7289, -1.5987) (19.7455, -1.5942) (19.7623, -1.5896) (19.779, -1.5849) (19.7959, -1.5801) (19.8128, -1.5753) (19.8297, -1.5705) (19.8468, -1.5655) (19.8639, -1.5605) (19.881, -1.5554) (19.8983, -1.5503) (19.9155, -1.5451) (19.9329, -1.5398) (19.9503, -1.5345) (19.9677, -1.5291) (19.9853, -1.5237) (20.0028, -1.5181) (20.0205, -1.5125) (20.0382, -1.5069) (20.0559, -1.5012) (20.0737, -1.4954) (20.0916, -1.4895) (20.1095, -1.4836) (20.1275, -1.4776) (20.1455, -1.4715) (20.1636, -1.4654) (20.1817, -1.4592) (20.1999, -1.453) (20.2181, -1.4466) (20.2364, -1.4402) (20.2547, -1.4338) (20.2731, -1.4273) (20.2915, -1.4207) (20.31, -1.414) (20.3285, -1.4073) (20.3471, -1.4005) (20.3657, -1.3936) (20.3844, -1.3867) (20.4031, -1.3797) (20.4219, -1.3726) (20.4407, -1.3655) (20.4596, -1.3583) (20.4785, -1.351) (20.4974, -1.3436) (20.5164, -1.3362) (20.5354, -1.3288) (20.5545, -1.3212) (20.5736, -1.3136) (20.5928, -1.3059) (20.612, -1.2982) (20.6313, -1.2903) (20.6505, -1.2824) (20.6699, -1.2745) (20.6892, -1.2665) (20.7086, -1.2584) (20.7281, -1.2502) (20.7476, -1.242) (20.7671, -1.2337) (20.7866, -1.2253) (20.8062, -1.2169) (20.8259, -1.2083) (20.8455, -1.1998) (20.8653, -1.1911) (20.885, -1.1824) (20.9048, -1.1736) (20.9246, -1.1648) (20.9444, -1.1558) (20.9643, -1.1468) (20.9842, -1.1378) (21.0042, -1.1286) (21.0242, -1.1194) (21.0442, -1.1102) (21.0642, -1.1008) (21.0843, -1.0914) (21.1044, -1.0819) (21.1246, -1.0724) (21.1447, -1.0628) (21.1649, -1.0531) (21.1852, -1.0433) (21.2054, -1.0335) (21.2257, -1.0236) (21.246, -1.0136) (21.2664, -1.0036) (21.2868, -0.9935) (21.3072, -0.9833) (21.3276, -0.9731) (21.3481, -0.9627) (21.3686, -0.9524) (21.3891, -0.9419) (21.4096, -0.9314) (21.4302, -0.9208) (21.4508, -0.9101) (21.4714, -0.8994) (21.492, -0.8886) (21.5127, -0.8777) (21.5334, -0.8668) (21.5541, -0.8557) (21.5748, -0.8447) (21.5956, -0.8335) (21.6164, -0.8223) (21.6372, -0.811) (21.658, -0.7996) (21.6789, -0.7882) (21.6997, -0.7767) (21.7206, -0.7651) (21.7415, -0.7535) (21.7625, -0.7417) (21.7834, -0.73) (21.8044, -0.7181) (21.8254, -0.7062) (21.8464, -0.6942) (21.8674, -0.6821) (21.8885, -0.67) (21.9096, -0.6578) (21.9307, -0.6455) (21.9518, -0.6332) (21.9729, -0.6207) (21.994, -0.6083) (22.0152, -0.5957) (22.0364, -0.5831) (22.0575, -0.5704) (22.0788, -0.5576) (22.1, -0.5448) (22.1212, -0.5319) (22.1425, -0.5189) (22.1637, -0.5059) (22.185, -0.4928) (22.2063, -0.4796) (22.2234, -0.469) (22.2362, -0.461) (22.2447, -0.4557) (22.249, -0.453) knots 0 0 0 0 0 0 0.00416667 0.00833333 0.0125 0.01666667 0.02083333 0.025 0.02916667 0.03333333 0.0375 0.04166667 0.04583333 0.05 0.05416667 0.05833333 0.0625 0.06666667 0.07083333 0.075 0.07916667 0.08333333 0.0875 0.09166667 0.09583333 0.1 0.10416667 0.10833333 0.1125 0.11666667 0.12083333 0.125 0.12916667 0.13333333 0.1375 0.14166667 0.14583333 0.15 0.15416667 0.15833333 0.1625 0.16666667 0.17083333 0.175 0.17916667 0.18333333 0.1875 0.19166667 0.19583333 0.2 0.20416667 0.20833333 0.2125 0.21666667 0.22083333 0.225 0.22916667 0.23333333 0.2375 0.24166667 0.24583333 0.25 0.25416667 0.25833333 0.2625 0.26666667 0.27083333 0.275 0.27916667 0.28333333 0.2875 0.29166667 0.29583333 0.3 0.30416667 0.30833333 0.3125 0.31666667 0.32083333 0.325 0.32916667 0.33333333 0.3375 0.34166667 0.34583333 0.35 0.35416667 0.35833333 0.3625 0.36666667 0.37083333 0.375 0.37916667 0.38333333 0.3875 0.39166667 0.39583333 0.4 0.40416667 0.40833333 0.4125 0.41666667 0.42083333 0.425 0.42916667 0.43333333 0.4375 0.44166667 0.44583333 0.45 0.45416667 0.45833333 0.4625 0.46666667 0.47083333 0.475 0.47916667 0.48333333 0.4875 0.49166667 0.49583333 0.5 0.50416667 0.50833333 0.5125 0.51666667 0.52083333 0.525 0.52916667 0.53333333 0.5375 0.54166667 0.54583333 0.55 0.55416667 0.55833333 0.5625 0.56666667 0.57083333 0.575 0.57916667 0.58333333 0.5875 0.59166667 0.59583333 0.6 0.60416667 0.60833333 0.6125 0.61666667 0.62083333 0.625 0.62916667 0.63333333 0.6375 0.64166667 0.64583333 0.65 0.65416667 0.65833333 0.6625 0.66666667 0.67083333 0.675 0.67916667 0.68333333 0.6875 0.69166667 0.69583333 0.7 0.70416667 0.70833333 0.7125 0.71666667 0.72083333 0.725 0.72916667 0.73333333 0.7375 0.74166667 0.74583333 0.75 0.75416667 0.75833333 0.7625 0.76666667 0.77083333 0.775 0.77916667 0.78333333 0.7875 0.79166667 0.79583333 0.8 0.80416667 0.80833333 0.8125 0.81666667 0.82083333 0.825 0.82916667 0.83333333 0.8375 0.84166667 0.84583333 0.85 0.85416667 0.85833333 0.8625 0.86666667 0.87083333 0.875 0.87916667 0.88333333 0.8875 0.89166667 0.89583333 0.9 0.90416667 0.90833333 0.9125 0.91666667 0.92083333 0.925 0.92916667 0.93333333 0.9375 0.94166667 0.94583333 0.95 0.95416667 0.95833333 0.9625 0.96666667 0.97083333 0.975 0.97916667 0.98333333 0.9875 0.99166667 0.99583333 1 1 1 1 1 1
  spline S1 degree 5 poles (18.5341, 1.774) (18.5343, 1.774) (18.5348, 1.7741) (18.5356, 1.7741) (18.5368, 1.7742) (18.5386, 1.7743) (18.5407, 1.7745) (18.5432, 1.7746) (18.5459, 1.7748) (18.5489, 1.775) (18.5521, 1.7751) (18.5556, 1.7753) (18.5594, 1.7755) (18.5634, 1.7756) (18.5676, 1.7758) (18.5721, 1.7759) (18.5768, 1.776) (18.5818, 1.7762) (18.587, 1.7763) (18.5924, 1.7764) (18.598, 1.7764) (18.6038, 1.7765) (18.6098, 1.7765) (18.616, 1.7766) (18.6224, 1.7765) (18.629, 1.7765) (18.6358, 1.7765) (18.6428, 1.7764) (18.65, 1.7763) (18.6574, 1.7761) (18.6649, 1.776) (18.6726, 1.7758) (18.6805, 1.7755) (18.6885, 1.7753) (18.6968, 1.775) (18.7051, 1.7747) (18.7137, 1.7743) (18.7224, 1.7739) (18.7313, 1.7735) (18.7403, 1.773) (18.7495, 1.7725) (18.7588, 1.7719) (18.7683, 1.7713) (18.7779, 1.7707) (18.7876, 1.77) (18.7975, 1.7693) (18.8076, 1.7686) (18.8178, 1.7678) (18.8281, 1.7669) (18.8386, 1.766) (18.8492, 1.7651) (18.8599, 1.7641) (18.8707, 1.7631) (18.8817, 1.762) (18.8928, 1.7609) (18.9041, 1.7598) (18.9154, 1.7586) (18.9269, 1.7573) (18.9385, 1.756) (18.9502, 1.7546) (18.9621, 1.7532) (18.974, 1.7518) (18.9861, 1.7503) (18.9983, 1.7487) (19.0106, 1.7471) (19.023, 1.7454) (19.0355, 1.7437) (19.0481, 1.742) (19.0609, 1.7401) (19.0737, 1.7383) (19.0867, 1.7363) (19.0997, 1.7344) (19.1129, 1.7323) (19.1261, 1.7302) (19.1395, 1.7281) (19.1529, 1.7259) (19.1665, 1.7237) (19.1801, 1.7213) (19.1939, 1.719) (19.2077, 1.7166) (19.2217, 1.7141) (19.2357, 1.7115) (19.2498, 1.7089) (19.2641, 1.7063) (19.2784, 1.7036) (19.2928, 1.7008) (19.3072, 1.698) (19.3218, 1.6951) (19.3365, 1.6921) (19.3512, 1.6891) (19.3661, 1.6861) (19.381, 1.683) (19.396, 1.6798) (19.4111, 1.6765) (19.4262, 1.6732) (19.4415, 1.6699) (19.4568, 1.6664) (19.4722, 1.663) (19.4877, 1.6594) (19.5033, 1.6558) (19.5189, 1.6521) (19.5346, 1.6484) (19.5504, 1.6446) (19.5663, 1.6407) (19.5822, 1.6368) (19.5982, 1.6328) (19.6143, 1.6288) (19.6305, 1.6247) (19.6467, 1.6205) (19.663, 1.6163) (19.6794, 1.612) (19.6958, 1.6076) (19.7123, 1.6032) (19.7289, 1.5987) (19.7455, 1.5942) (19.7623, 1.5896) (19.779, 1.5849) (19.7959, 1.5801) (19.8128, 1.5753) (19.8297, 1.5705) (19.8468, 1.5655) (19.8639, 1.5605) (19.881, 1.5554) (19.8983, 1.5503) (19.9155, 1.5451) (19.9329, 1.5398) (19.9503, 1.5345) (19.9677, 1.5291) (19.9853, 1.5237) (20.0028, 1.5181) (20.0205, 1.5125) (20.0382, 1.5069) (20.0559, 1.5012) (20.0737, 1.4954) (20.0916, 1.4895) (20.1095, 1.4836) (20.1275, 1.4776) (20.1455, 1.4715) (20.1636, 1.4654) (20.1817, 1.4592) (20.1999, 1.453) (20.2181, 1.4466) (20.2364, 1.4402) (20.2547, 1.4338) (20.2731, 1.4273) (20.2915, 1.4207) (20.31, 1.414) (20.3285, 1.4073) (20.3471, 1.4005) (20.3657, 1.3936) (20.3844, 1.3867) (20.4031, 1.3797) (20.4219, 1.3726) (20.4407, 1.3655) (20.4596, 1.3583) (20.4785, 1.351) (20.4974, 1.3436) (20.5164, 1.3362) (20.5354, 1.3288) (20.5545, 1.3212) (20.5736, 1.3136) (20.5928, 1.3059) (20.612, 1.2982) (20.6313, 1.2903) (20.6505, 1.2824) (20.6699, 1.2745) (20.6892, 1.2665) (20.7086, 1.2584) (20.7281, 1.2502) (20.7476, 1.242) (20.7671, 1.2337) (20.7866, 1.2253) (20.8062, 1.2169) (20.8259, 1.2083) (20.8455, 1.1998) (20.8653, 1.1911) (20.885, 1.1824) (20.9048, 1.1736) (20.9246, 1.1648) (20.9444, 1.1558) (20.9643, 1.1468) (20.9842, 1.1378) (21.0042, 1.1286) (21.0242, 1.1194) (21.0442, 1.1102) (21.0642, 1.1008) (21.0843, 1.0914) (21.1044, 1.0819) (21.1246, 1.0724) (21.1447, 1.0628) (21.1649, 1.0531) (21.1852, 1.0433) (21.2054, 1.0335) (21.2257, 1.0236) (21.246, 1.0136) (21.2664, 1.0036) (21.2868, 0.9935) (21.3072, 0.9833) (21.3276, 0.9731) (21.3481, 0.9627) (21.3686, 0.9524) (21.3891, 0.9419) (21.4096, 0.9314) (21.4302, 0.9208) (21.4508, 0.9101) (21.4714, 0.8994) (21.492, 0.8886) (21.5127, 0.8777) (21.5334, 0.8668) (21.5541, 0.8557) (21.5748, 0.8447) (21.5956, 0.8335) (21.6164, 0.8223) (21.6372, 0.811) (21.658, 0.7996) (21.6789, 0.7882) (21.6997, 0.7767) (21.7206, 0.7651) (21.7415, 0.7535) (21.7625, 0.7417) (21.7834, 0.73) (21.8044, 0.7181) (21.8254, 0.7062) (21.8464, 0.6942) (21.8674, 0.6821) (21.8885, 0.67) (21.9096, 0.6578) (21.9307, 0.6455) (21.9518, 0.6332) (21.9729, 0.6207) (21.994, 0.6083) (22.0152, 0.5957) (22.0364, 0.5831) (22.0575, 0.5704) (22.0788, 0.5576) (22.1, 0.5448) (22.1212, 0.5319) (22.1425, 0.5189) (22.1637, 0.5059) (22.185, 0.4928) (22.2063, 0.4796) (22.2234, 0.469) (22.2362, 0.461) (22.2447, 0.4557) (22.249, 0.453) knots 0 0 0 0 0 0 0.00416667 0.00833333 0.0125 0.01666667 0.02083333 0.025 0.02916667 0.03333333 0.0375 0.04166667 0.04583333 0.05 0.05416667 0.05833333 0.0625 0.06666667 0.07083333 0.075 0.07916667 0.08333333 0.0875 0.09166667 0.09583333 0.1 0.10416667 0.10833333 0.1125 0.11666667 0.12083333 0.125 0.12916667 0.13333333 0.1375 0.14166667 0.14583333 0.15 0.15416667 0.15833333 0.1625 0.16666667 0.17083333 0.175 0.17916667 0.18333333 0.1875 0.19166667 0.19583333 0.2 0.20416667 0.20833333 0.2125 0.21666667 0.22083333 0.225 0.22916667 0.23333333 0.2375 0.24166667 0.24583333 0.25 0.25416667 0.25833333 0.2625 0.26666667 0.27083333 0.275 0.27916667 0.28333333 0.2875 0.29166667 0.29583333 0.3 0.30416667 0.30833333 0.3125 0.31666667 0.32083333 0.325 0.32916667 0.33333333 0.3375 0.34166667 0.34583333 0.35 0.35416667 0.35833333 0.3625 0.36666667 0.37083333 0.375 0.37916667 0.38333333 0.3875 0.39166667 0.39583333 0.4 0.40416667 0.40833333 0.4125 0.41666667 0.42083333 0.425 0.42916667 0.43333333 0.4375 0.44166667 0.44583333 0.45 0.45416667 0.45833333 0.4625 0.46666667 0.47083333 0.475 0.47916667 0.48333333 0.4875 0.49166667 0.49583333 0.5 0.50416667 0.50833333 0.5125 0.51666667 0.52083333 0.525 0.52916667 0.53333333 0.5375 0.54166667 0.54583333 0.55 0.55416667 0.55833333 0.5625 0.56666667 0.57083333 0.575 0.57916667 0.58333333 0.5875 0.59166667 0.59583333 0.6 0.60416667 0.60833333 0.6125 0.61666667 0.62083333 0.625 0.62916667 0.63333333 0.6375 0.64166667 0.64583333 0.65 0.65416667 0.65833333 0.6625 0.66666667 0.67083333 0.675 0.67916667 0.68333333 0.6875 0.69166667 0.69583333 0.7 0.70416667 0.70833333 0.7125 0.71666667 0.72083333 0.725 0.72916667 0.73333333 0.7375 0.74166667 0.74583333 0.75 0.75416667 0.75833333 0.7625 0.76666667 0.77083333 0.775 0.77916667 0.78333333 0.7875 0.79166667 0.79583333 0.8 0.80416667 0.80833333 0.8125 0.81666667 0.82083333 0.825 0.82916667 0.83333333 0.8375 0.84166667 0.84583333 0.85 0.85416667 0.85833333 0.8625 0.86666667 0.87083333 0.875 0.87916667 0.88333333 0.8875 0.89166667 0.89583333 0.9 0.90416667 0.90833333 0.9125 0.91666667 0.92083333 0.925 0.92916667 0.93333333 0.9375 0.94166667 0.94583333 0.95 0.95416667 0.95833333 0.9625 0.96666667 0.97083333 0.975 0.97916667 0.98333333 0.9875 0.99166667 0.99583333 1 1 1 1 1 1
  spline S2 degree 5 poles (18.5324, -1.7738) (18.5325, -1.7739) (18.5326, -1.7739) (18.5328, -1.7739) (18.5331, -1.7739) (18.5334, -1.7739) (18.5337, -1.774) (18.5339, -1.774) (18.534, -1.774) (18.5341, -1.774) knots 0 0 0 0 0 0 0.2 0.4 0.6 0.8 1 1 1 1 1 1
  spline S3 degree 5 poles (18.5324, 1.7738) (18.5325, 1.7739) (18.5326, 1.7739) (18.5328, 1.7739) (18.5331, 1.7739) (18.5334, 1.7739) (18.5337, 1.774) (18.5339, 1.774) (18.534, 1.774) (18.5341, 1.774) knots 0 0 0 0 0 0 0.2 0.4 0.6 0.8 1 1 1 1 1 1
  line L0 (0, 0) -> (18.5324, -1.7738)
  line L1 (0, 0) -> (18.5324, 1.7738)
  arc A0 (22.249, -0.453) -> (22.249, 0.453) centre (0, 0) ccw
  point P0 (18.5391, -1.7744)
  point P1 (18.5474, -1.7749)
  point P2 (18.559, -1.7754)
  point P3 (18.574, -1.776)
  point P4 (18.5922, -1.7764)
  point P5 (18.6138, -1.7765)
  point P6 (18.6388, -1.7764)
  point P7 (18.667, -1.7759)
  point P8 (18.6986, -1.7749)
  point P9 (18.7335, -1.7733)
  point P10 (18.7717, -1.7711)
  point P11 (18.8131, -1.7681)
  point P12 (18.8578, -1.7643)
  point P13 (18.9058, -1.7596)
  point P14 (18.957, -1.7538)
  point P15 (19.0115, -1.747)
  point P16 (19.0691, -1.7389)
  point P17 (19.1299, -1.7296)
  point P18 (19.1938, -1.719)
  point P19 (19.2609, -1.7069)
  point P20 (19.3311, -1.6932)
  point P21 (19.4043, -1.678)
  point P22 (19.4806, -1.661)
  point P23 (19.5599, -1.6423)
  point P24 (19.6421, -1.6217)
  point P25 (19.7273, -1.5991)
  point P26 (19.8154, -1.5746)
  point P27 (19.9063, -1.5479)
  point P28 (20, -1.519)
  point P29 (20.0965, -1.4879)
  point P30 (20.1958, -1.4544)
  point P31 (20.2977, -1.4184)
  point P32 (20.4022, -1.38)
  point P33 (20.5093, -1.339)
  point P34 (20.619, -1.2953)
  point P35 (20.7311, -1.2489)
  point P36 (20.8457, -1.1997)
  point P37 (20.9626, -1.1476)
  point P38 (21.0819, -1.0926)
  point P39 (21.2034, -1.0345)
  point P40 (21.3271, -0.9733)
  point P41 (21.4529, -0.909)
  point P42 (21.5808, -0.8415)
  point P43 (21.7107, -0.7706)
  point P44 (21.8425, -0.6964)
  point P45 (21.9762, -0.6188)
  point P46 (22.1117, -0.5377)
  point P47 (18.5391, 1.7744)
  point P48 (18.5474, 1.7749)
  point P49 (18.559, 1.7754)
  point P50 (18.574, 1.776)
  point P51 (18.5922, 1.7764)
  point P52 (18.6138, 1.7765)
  point P53 (18.6388, 1.7764)
  point P54 (18.667, 1.7759)
  point P55 (18.6986, 1.7749)
  point P56 (18.7335, 1.7733)
  point P57 (18.7717, 1.7711)
  point P58 (18.8131, 1.7681)
  point P59 (18.8578, 1.7643)
  point P60 (18.9058, 1.7596)
  point P61 (18.957, 1.7538)
  point P62 (19.0115, 1.747)
  point P63 (19.0691, 1.7389)
  point P64 (19.1299, 1.7296)
  point P65 (19.1938, 1.719)
  point P66 (19.2609, 1.7069)
  point P67 (19.3311, 1.6932)
  point P68 (19.4043, 1.678)
  point P69 (19.4806, 1.661)
  point P70 (19.5599, 1.6423)
  point P71 (19.6421, 1.6217)
  point P72 (19.7273, 1.5991)
  point P73 (19.8154, 1.5746)
  point P74 (19.9063, 1.5479)
  point P75 (20, 1.519)
  point P76 (20.0965, 1.4879)
  point P77 (20.1958, 1.4544)
  point P78 (20.2977, 1.4184)
  point P79 (20.4022, 1.38)
  point P80 (20.5093, 1.339)
  point P81 (20.619, 1.2953)
  point P82 (20.7311, 1.2489)
  point P83 (20.8457, 1.1997)
  point P84 (20.9626, 1.1476)
  point P85 (21.0819, 1.0926)
  point P86 (21.2034, 1.0345)
  point P87 (21.3271, 0.9733)
  point P88 (21.4529, 0.909)
  point P89 (21.5808, 0.8415)
  point P90 (21.7107, 0.7706)
  point P91 (21.8425, 0.6964)
  point P92 (21.9762, 0.6188)
  point P93 (22.1117, 0.5377)
sketch "Sketch2 (2)" plane through (0, 0, 0) normal (0, 0, 1) x (1, 0, 0) in component "Component'"
  circle A0 centre (0, 0) radius 18.402
extrude "Extrude1'" add sketch "Sketch2 (2)" along normal blind 3 separate body makes body 10 in component "Component'"
extrude "Extrude2'" add sketch "Sketch1 (2)" along normal blind 3 separate body makes body 11 in component "Component'"
pattern_circular "C-Pattern1'" count 24 over 360 about axis through (0, 0, 1.75) along (0, 0, 1) of "Extrude2'" makes body 12 at (5.8145, 2.1702, 1) makes body 13 at (5.646, 2.5769, 1) makes body 14 at (4.7867, 3.9504, 1) makes body 15 at (3.6011, 5.0547, 1) makes body 16 at (1.0278, 6.1206, 1) makes body 17 at (0.5913, 6.178, 1) makes body 18 at (-1.0278, 6.1206, 1) makes body 19 at (-3.6011, 5.0547, 1) makes body 20 at (-3.9504, 4.7867, 1) makes body 21 at (-5.0547, 3.6011, 1) makes body 22 at (-5.8145, 2.1702, 2) makes body 23 at (-6.178, 0.5913, 1) makes body 24 at (-6.1206, -1.0278, 1) makes body 25 at (-5.646, -2.5769, 1) makes body 26 at (-4.7867, -3.9504, 1) makes body 27 at (-3.6011, -5.0547, 1) makes body 28 at (-1.0278, -6.1206, 1) makes body 29 at (-0.5913, -6.178, 1) makes body 30 at (1.0278, -6.1206, 1) makes body 31 at (2.5769, -5.646, 1) makes body 32 at (3.9504, -4.7867, 1) makes body 33 at (5.0547, -3.6011, 1) makes body 34 at (5.8145, -2.1702, 1) in component "Component'"
combine "Combine1'" operation add target body 10 tool bodies 11 12 13 14 15 16 17 18 19 20 21 22 23 24 25 26 27 28 29 30 31 32 33 34 in component "Component'"
sketch "Sketch3 (2)" plane through (0, 0, 0) normal (0, 0, 1) x (1, 0, 0) in component "Component'"
  line L0 (0, 0) -> (52.5498, 0) construction
  line L1 (52.5498, 0) -> (52.5498, 3) construction
  line L2 (52.5498, 3) -> (0, 3) construction
  line L3 (0, 3) -> (0, 0) construction
  constraint perpendicular L0 L1
  constraint parallel L0 L2
  constraint parallel L1 L3